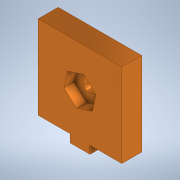
# Autodesk Inventor part: gaica cu suportul
Saved by Autodesk Inventor 2021.2 (Build 252289000, 289)
## iProperties
Created: 2024-04-19
Part Number: gaica cu suportul
Material: Gold
Document SubType Name: Modeling
Designer: cioba
Density: 19.3 g/cm^3
Appearance: Metal 1600F Hot
Author: cioba
Autodesk Inventor part; units mm, degrees
ref_plane "YZ Plane" through (0, 0, 0) normal (1, 0, 0) x (0, 1, 0)
ref_plane "XZ Plane" through (0, 0, 0) normal (0, 1, 0) x (-1, 0, 0)
ref_plane "XY Plane" through (0, 0, 0) normal (0, 0, 1) x (1, 0, 0)
sketch "Sketch1" plane through (0, 0, 0) normal (0, 0, 1) x (1, 0, 0)
  line L0 (-8.9346, 3.531) -> (-24.9346, 3.531)
  line L1 (-24.9346, 3.531) -> (-24.9346, 45.531)
  line L2 (-24.9346, 45.531) -> (17.0654, 45.531)
  line L3 (17.0654, 45.531) -> (17.0654, 3.531)
  line L4 (17.0654, 3.531) -> (1.0654, 3.531)
  line L5 (4.0654, 27.1063) -> (2.3055, 18.8848)
  line L6 (2.3055, 18.8848) -> (-5.6945, 16.2981)
  line L7 (-5.6945, 16.2981) -> (-11.9346, 21.933)
  line L8 (-11.9346, 21.933) -> (-10.1748, 30.1545)
  line L9 (-10.1748, 30.1545) -> (-2.1748, 32.7412)
  line L10 (-2.1748, 32.7412) -> (4.0654, 27.1063)
  circle A0 centre (-3.9346, 24.5196) radius 3.5
  line L11 (-8.9346, -0.469) -> (1.0654, -0.469)
  line L12 (-8.9346, 3.531) -> (-8.9346, -0.469)
  line L13 (1.0654, 3.531) -> (1.0654, -0.469)
  point P0 (0, 0)
  constraints: 28 end point, 2 perpendicular, 2 point on line, 1 centre point, 1 coincident, 1 parallel, 1 vertical, 13 other
extrude "Extrusion1" add sketch "Sketch1" against normal blind 10 contours L0 L1 L2 L3 L4 L13 L11 L12 | L5 L6 L7 L8 L9 L10 | A0
extrude "Extrusion2" cut sketch "Sketch1" against normal through all contours A0
extrude "Extrusion3" cut sketch "Sketch1" against normal blind 5 contours L5 L6 L7 L8 L9 L10
body "Solid1"
